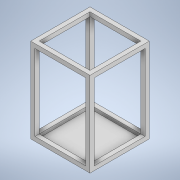
# Autodesk Inventor part: Frame
Saved by Autodesk Inventor 2022 (Build 260153000, 153)
## iProperties
Created: 2021-06-22
Part Number: Frame
Material: Generic
Document SubType Name: Modeling
Designer: Admin
Density: 1 g/cm^3
Appearance: Default
Author: Admin
Autodesk Inventor part; units mm, degrees
ref_plane "YZ Plane" through (0, 0, 0) normal (1, 0, 0) x (0, 1, 0)
ref_plane "XZ Plane" through (0, 0, 0) normal (0, 1, 0) x (-1, 0, 0)
ref_plane "XY Plane" through (0, 0, 0) normal (0, 0, 1) x (1, 0, 0)
sketch "Sketch1" plane through (0, 0, 0) normal (0, 0, 1) x (1, 0, 0)
  point P0 (0, 0)
sketch "Sketch2" plane through (0, 0, 0) normal (0, 1, 0) x (-1, 0, 0)
  line L0 (-300, 300) -> (300, 300)
  line L1 (300, 300) -> (300, -300)
  line L2 (300, -300) -> (-300, -300)
  line L3 (-300, -300) -> (-300, 300)
  line L4 (-300, 300) -> (300, -300) construction
  line L5 (300, 300) -> (-300, -300) construction
  line L6 (350, 350) -> (-350, 350)
  line L7 (-350, 350) -> (-350, -350)
  line L8 (-350, -350) -> (350, -350)
  line L9 (350, -350) -> (350, 350)
  line L10 (350, 350) -> (-350, -350) construction
  line L11 (-350, 350) -> (350, -350) construction
  line L12 (-300, 300) -> (-350, 300)
  line L13 (-350, 300) -> (-350, 350)
  line L14 (-350, 350) -> (-300, 350)
  line L15 (-300, 350) -> (-300, 300)
  line L16 (300, 300) -> (350, 300)
  line L17 (350, 300) -> (350, 350)
  line L18 (350, 350) -> (300, 350)
  line L19 (300, 350) -> (300, 300)
  line L20 (350, -350) -> (300, -350)
  line L21 (300, -350) -> (300, -300)
  line L22 (300, -300) -> (350, -300)
  line L23 (350, -300) -> (350, -350)
  line L24 (-350, -350) -> (-300, -350)
  line L25 (-300, -350) -> (-300, -300)
  line L26 (-300, -300) -> (-350, -300)
  line L27 (-350, -300) -> (-350, -350)
  point P0 (0, 0)
  dimension "d0" = 600
  dimension "d1" = 600
  dimension "d2" = 700
  dimension "d3" = 700
  constraints: 56 end point, 12 parallel, 6 horizontal, 6 perpendicular, 4 midpoint
  measures "d0" distance of L1.end L2.end
  measures "d1" distance of L0.end L1.end
  measures "d2" distance of L8.end L7.end
  measures "d3" distance of L7.end L6.end
extrude "Extrusion1" add sketch "Sketch2" along normal blind 10 contours L0 L1 L2 L3
extrude "Extrusion2" add sketch "Sketch2" along normal blind 50 contours L15 L6 L19 L0 | L3 L26 L7 L12 | L12 L7 L6 L15 | L16 L9 L22 L1 | L19 L6 L9 L16 | L2 L21 L8 L25 | L25 L8 L7 L26 | L22 L9 L8 L21
extrude "Extrusion3" add sketch "Sketch2" along normal blind 1000 contours L12 L7 L6 L15 | L19 L6 L9 L16 | L25 L8 L7 L26 | L22 L9 L8 L21
sketch3d "3D Sketch1"
sketch "Sketch3" plane through (-300, 50, 300) normal (1, 0, 0) x (0, 0, -1)
  line L0 (-50, -50) -> (-50, 950) projected
  line L1 (0, 0) -> (0, 950) projected
  line L2 (-50, 950) -> (0, 950)
  line L3 (0, 950) -> (0, 900)
  line L4 (0, 900) -> (-50, 900)
  line L5 (-50, 900) -> (-50, 950)
  point P0 (300, -50)
  dimension "d13" = 50
  constraints: 8 end point, 2 parallel, 1 horizontal, 1 perpendicular, 1 point on line
  measures "d13" distance of L2.end L3.end
sketch "Sketch4" plane through (-300, 50, 300) normal (1, 0, 0) x (0, 0, -1)
  point P0 (300, -50)
extrude "Extrusion4" add sketch "Sketch3" along normal up to surface (600 mm away)
sketch "Sketch5" plane through (300, 50, -300) normal (0, 0, 1) x (1, 0, 0)
  line L0 (50, 950) -> (-650, 950) projected
  line L1 (0, 0) -> (0, 900) projected
  line L2 (50, 950) -> (0, 950)
  line L3 (0, 950) -> (0, 900)
  line L4 (0, 900) -> (50, 900)
  line L5 (50, 900) -> (50, 950)
  point P0 (-300, -50)
  constraints: 8 end point, 2 parallel, 1 horizontal, 1 perpendicular
extrude "Extrusion5" add sketch "Sketch5" along normal up to surface (600 mm away)
sketch "Sketch6" plane through (-300, 50, -350) normal (1, 0, 0) x (0, 0, -1)
  line L0 (-50, 0) -> (-50, 950) projected
  line L1 (0, 0) -> (0, 950) projected
  line L2 (-50, 950) -> (0, 950)
  line L3 (0, 950) -> (0, 900)
  line L4 (0, 900) -> (-50, 900)
  line L5 (-50, 900) -> (-50, 950)
  point P0 (-350, -50)
  dimension "d18" = 50
  constraints: 8 end point, 2 parallel, 1 horizontal, 1 perpendicular, 1 point on line
  measures "d18" distance of L2.end L3.end
extrude "Extrusion6" add sketch "Sketch6" along normal up to surface (600 mm away)
sketch "Sketch7" plane through (-350, 1000, -300) normal (0, 0, 1) x (1, 0, 0)
  line L0 (0, -950) -> (0, 0) projected
  line L1 (50, -950) -> (50, -50) projected
  line L2 (0, 0) -> (50, 0)
  line L3 (50, 0) -> (50, -50)
  line L4 (50, -50) -> (0, -50)
  line L5 (0, -50) -> (0, 0)
  point P0 (350, -1000)
  constraints: 8 end point, 2 parallel, 1 horizontal, 1 perpendicular
extrude "Extrusion7" add sketch "Sketch7" along normal up to surface (600 mm away)
body "Solid1"
